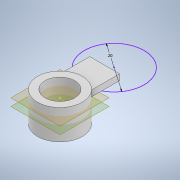
# Autodesk Inventor part: KEP_BUT
Saved by Autodesk Inventor 2022 (Build 260153000, 153)
## iProperties
Created: 2022-11-18
Part Number: KEP_BUT
Material: Generic
Document SubType Name: Modeling
Designer: nguye
Density: 1 g/cm^3
Appearance: Default
Author: nguye
Autodesk Inventor part; units mm, degrees
ref_plane "YZ Plane" through (0, 0, 0) normal (1, 0, 0) x (0, 1, 0)
ref_plane "XZ Plane" through (0, 0, 0) normal (0, 1, 0) x (-1, 0, 0)
ref_plane "XY Plane" through (0, 0, 0) normal (0, 0, 1) x (1, 0, 0)
sketch "Sketch1" plane through (0, 0, 0) normal (0, 1, 0) x (-1, 0, 0)
  circle A0 centre (0, 0) radius 5
  circle A1 centre (0, 0) radius 7.5
  dimension "d0" = 10
  dimension "d1" = 15
  constraints: 2 centre point, 2 coincident
  measures "d0" diameter of A0
  measures "d1" diameter of A1
extrude "Extrusion1" add sketch "Sketch1" along normal blind 10
ref_plane "Work Plane1" through (0, 7.5, 0) normal (0, 1, 0) x (1, 0, 0)
sketch "Sketch2" plane through (0, 7.5, 0) normal (0, 1, 0) x (1, 0, 0)
  line L0 (-5, 5.5902) -> (-5, 15)
  line L1 (-5, 15) -> (5, 15)
  line L2 (5, 15) -> (5, 5.5902)
  circle A0 centre (0, 0) radius 7.5 projected
  circle A1 centre (0, 0) radius 7.5 projected
  dimension "d5" = 10
  dimension "d6" = 5
  dimension "d7" = 15
  constraints: 6 end point, 2 perpendicular, 1 point on circle, 1 vertical, 2 other
  measures "d5" distance of L0.end L1.end
  measures "d6" distance from line of point (0, 0) L0
  measures "d7" distance from line of point (0, 0) L1
extrude "Extrusion2" add sketch "Sketch2" along normal blind 2 contours L0 L1 L2 A0
ref_plane "Work Plane2" through (0, 5, 0) normal (0, -1, 0) x (1, 0, 0)
sketch "Sketch4" plane through (0, 7.5, 0) normal (0, -1, 0) x (1, 0, 0)
  circle A0 centre (0.2579, -17.9126) radius 10
  point P0 (0, 0)
  dimension "d11" = 20
  constraints: 1 centre point
  measures "d11" diameter of A0
body "Solid1"
